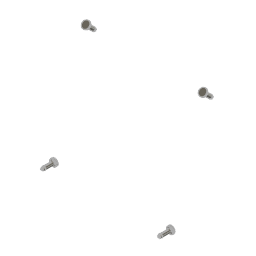
Fusion_native_pin_assembly (Autodesk Fusion 360 design; units mm, degrees)
Autodesk Fusion 360 part; units mm, degrees
sketch "Pin - dimensioned axial profile" plane through (0, 0, 0) normal (0, 1, 0) x (1, 0, 0) in component "Push pin - native"
  line L0 (0, 0) -> (4, 0)
  line L1 (4, 0) -> (4, -1.4)
  line L2 (4, -1.4) -> (3.4, -2)
  line L3 (3.4, -2) -> (2, -2)
  line L4 (2, -2) -> (2, -12)
  line L5 (2, -12) -> (2.1, -12)
  line L6 (2.1, -12) -> (1.6, -14)
  line L7 (1.6, -14) -> (0, -14)
  line L8 (0, -14) -> (0, 0)
  dimension "d12" = 4
  dimension "d13" = 1.4
  dimension "d14" = 0.8485
  dimension "d15" = 1.4
  dimension "d16" = 10
  dimension "d17" = 0.1
  dimension "d18" = 2.0616
  dimension "d19" = 1.6
  dimension "d20" = 14
  constraint horizontal L0
  constraint vertical L1
  constraint horizontal L3
  constraint vertical L4
  constraint horizontal L5
  constraint horizontal L7
  constraint vertical L8
  measures "d12" distance of L0.start L0.end
  measures "d13" distance of L0.end L1.end
  measures "d14" distance of L1.end L2.end
  measures "d15" distance of L2.end L3.end
  measures "d16" distance of L3.end L4.end
  measures "d17" distance of L4.end L5.end
  measures "d18" distance of L5.end L6.end
  measures "d19" distance of L6.end L7.end
  measures "d20" distance of L0.start L7.end
revolve "Pin - full revolve" add sketch "Pin - dimensioned axial profile" angle 360 about axis through (0, 0, 14) along (0, 0, -1) in component "Push pin - native"
sketch "Pin - split profile" plane through (0, 0, 0) normal (0, 1, 0) x (1, 0, 0) in component "Push pin - native"
  line L0 (-0.5, -4) -> (0.5, -4)
  line L1 (0.5, -4) -> (0.5, -14.1)
  line L2 (0.5, -14.1) -> (-0.5, -14.1)
  line L3 (-0.5, -14.1) -> (-0.5, -4)
  dimension "d22" = 1
  dimension "d23" = 10.1
  measures "d22" distance of L0.start L0.end
  measures "d23" distance of L0.end L1.end
extrude "Pin - symmetric split cut" cut sketch "Pin - split profile" along normal mid plane 6 in component "Push pin - native"
component "Push pin - native" placed x (1, 0, 0) y (0, 1, 0) z (0, 0, 1) at (0, 0, 0)
component "Push pin - native" placed x (1, 0, 0) y (0, 1, 0) z (0, 0, 1) at (130, 0, 0)
component "Push pin - native" placed x (1, 0, 0) y (0, -0.707107, 0.707107) z (0, -0.707107, -0.707107) at (5, 120.033, -29.5528)
component "Push pin - native" placed x (1, 0, 0) y (0, -0.707107, 0.707107) z (0, -0.707107, -0.707107) at (135, 120.033, -29.5528)
equation "pinHeadRadius = 4 mm" comment "Revision F pin"
equation "pinHeadHeight = 2 mm" comment "Revision F pin"
equation "pinHeadChamfer = 0.6 mm" comment "Revision F pin"
equation "pinShaftDiameter = 4 mm" comment "Revision F pin"
equation "pinShaftLength = 10 mm" comment "Revision F pin"
equation "pinCrownDiameter = 4.2 mm" comment "Revision F pin"
equation "pinCrownHeight = 2 mm" comment "Revision F pin"
equation "pinTipRadius = 1.6 mm" comment "Revision F pin"
equation "pinSplitWidth = 1 mm" comment "Revision F pin"
equation "pinSplitRoot = 4 mm" comment "Revision F pin"
equation "pinSplitOverrun = 0.1 mm" comment "Revision F pin"
equation "d12 = pinHeadRadius"
equation "d13 = pinHeadHeight - pinHeadChamfer"
equation "d14 = sqrt(2) * pinHeadChamfer"
equation "d15 = pinHeadRadius - pinHeadChamfer - pinShaftDiameter / 2"
equation "d16 = pinShaftLength"
equation "d17 = ( pinCrownDiameter - pinShaftDiameter ) / 2"
equation "d18 = sqrt(( pinCrownDiameter / 2 - pinTipRadius ) ^ 2 + pinCrownHeight ^ 2)"
equation "d19 = pinTipRadius"
equation "d20 = pinHeadHeight + pinShaftLength + pinCrownHeight"
equation "d22 = pinSplitWidth"
equation "d23 = pinHeadHeight + pinShaftLength + pinCrownHeight + pinSplitOverrun - pinSplitRoot"
named bodies: "Revision F split push pin"
